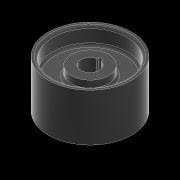
# Autodesk Inventor part: WheelHubMockup
Saved by Autodesk Inventor 2021 (Build 250183000, 183)
## iProperties
Created: 2021-03-11
Part Number: WheelHubMockup
Material: Nylon 6/6
Document SubType Name: Modeling
Designer: Esketitttttt
Density: 1.13 g/cm^3
Appearance: Matteee Blackkkk Default Plastic
Mass: 408.743 g
Surface Area: 695.671 cm^2
Volume: 361.72 cm^3
Author: Esketitttttt
Autodesk Inventor part; units mm, degrees
ref_plane "YZ Plane" through (0, 0, 0) normal (1, 0, 0) x (0, 1, 0)
ref_plane "XZ Plane" through (0, 0, 0) normal (0, 1, 0) x (-1, 0, 0)
sketch "Sketch1" plane through (0, 0, 0) normal (0, 1, 0) x (-1, 0, 0)
  circle A0 centre (0, 0) radius 12.7127
  circle A1 centre (0, 0) radius 12.7127
  line L0 (3.175, -12.3098) -> (3.175, -15.4848)
  line L1 (3.175, -15.4848) -> (-3.175, -15.4848)
  line L2 (-3.175, -12.3098) -> (-3.175, -15.4848)
  circle A2 centre (0, 0) radius 25.4
  circle A3 centre (0, 0) radius 50.8
  circle A4 centre (0, 0) radius 57.15
  point P0 (0, -12.7127)
  dimension "d0" = 3.175
  dimension "d1" = 50.8
  dimension "d6" = 101.6
  dimension "d7" = 6.35
  constraints: 6 end point, 5 centre point, 3 point on circle, 2 coincident
  measures "d0" distance of L0.start L0.end
  measures "d1" diameter of A2
  measures "d6" diameter of A3
  measures "d7" radial gap between concentric circles of A3 A4
extrude "BaseKeying" add sketch "Sketch1" along normal blind 63.5 contours A2
extrude "ExtraSpacing" add sketch "Sketch1" against normal blind 6.35 contours A2
ref_plane "Work Plane1" through (0, 44.45, 0) normal (0, 1, 0) x (1, 0, 0)
sketch "Sketch2" plane through (0, 44.45, 0) normal (0, 1, 0) x (1, 0, 0)
  circle A0 centre (0, 0) radius 50.8 projected
  circle A1 centre (0, 0) radius 25.4 projected
extrude "MidPart" add sketch "Sketch2" along normal blind 6.35 and the other way blind 12.7
sketch "Sketch3" plane through (0, 44.45, 0) normal (0, 1, 0) x (1, 0, 0)
  circle A0 centre (0, 0) radius 57.15 projected
  circle A1 centre (0, 0) radius 50.8 projected
extrude "OuterRing" add sketch "Sketch3" along normal blind 29.6333 and the other way blind 35.56
fillet "Fillet1" radius 3.175 6 edges at (25.4, 50.8, 0) (25.4, 31.75, 0) (-50.8, 31.75, 0) (-50.8, 8.89, 0) (-50.8, 50.8, 0) (-50.8, 74.0833, 0)
body "Solid1"
